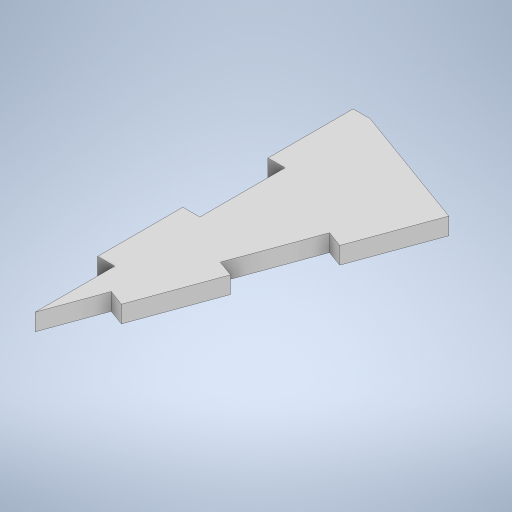
# Autodesk Inventor part: do_sensor_2
Saved by Autodesk Inventor 2023 (Build 270158000, 158)
## iProperties
Created: 2022-11-21
Part Number: do_sensor_2
Material: Generic
Document SubType Name: Modeling
Designer: ADMIN
Density: 1 g/cm^3
Appearance: Default
Author: ADMIN
Autodesk Inventor part; units mm, degrees
ref_plane "YZ Plane" through (0, 0, 0) normal (1, 0, 0) x (0, 1, 0)
ref_plane "XZ Plane" through (0, 0, 0) normal (0, 1, 0) x (-1, 0, 0)
ref_plane "XY Plane" through (0, 0, 0) normal (0, 0, 1) x (1, 0, 0)
sketch "Sketch1" plane through (0, 0, 0) normal (0, 1, 0) x (-1, 0, 0)
  line L0 (-13.5, -14) -> (-32.4622, -7.0983)
  line L1 (-13.5, -14) -> (-10.5, -14)
  line L2 (-10.5, -14) -> (-10.5, 1)
  line L3 (-10.5, 1) -> (-13.5, 1)
  line L4 (-13.5, 1) -> (-13.5, 16)
  line L5 (-13.5, 16) -> (-10.5, 16)
  line L6 (-10.5, 16) -> (-10.5, 31)
  line L7 (-10.5, 31) -> (-13.5, 31)
  line L8 (-13.5, 45) -> (-13.5, 31)
  line L9 (-13.5, 16) -> (-13.5, 1)
  line L10 (-32.4622, -7.0983) -> (-35.2813, -6.0723)
  line L11 (-35.2813, -6.0723) -> (-30.151, 8.0231)
  line L12 (-30.151, 8.0231) -> (-27.3319, 6.9971)
  line L13 (-27.3319, 6.9971) -> (-22.2016, 21.0925)
  line L14 (-22.2016, 21.0925) -> (-25.0207, 22.1185)
  line L15 (-25.0207, 22.1185) -> (-19.8904, 36.2139)
  line L16 (-19.8904, 36.2139) -> (-17.0713, 35.1879)
  line L17 (-13.5, 45) -> (-17.0713, 35.1879)
  line L18 (-22.2016, 21.0925) -> (-27.3319, 6.9971)
  point P0 (0, 0)
  dimension "d0" = 3
  dimension "d1" = 15
  dimension "d2" = 15
  dimension "d3" = 15
  dimension "d4" = 15
  dimension "d5" = 15
  dimension "d6" = 15
  dimension "d7" = 2.8191
  constraints: 38 end point, 14 perpendicular, 2 point on line, 1 vertical
  measures "d0" distance of L0.start L1.end
  measures "d1" distance of L1.end L3.start
  measures "d2" distance of L4.start L5.start
  measures "d3" distance of L5.end L7.start
  measures "d4" distance of L11.start L12.start
  measures "d5" distance of L13.start L14.start
  measures "d6" distance of L14.end L15.end
  measures "d7" horizontal distance of L12.start L13.start
extrude "Extrusion1" add sketch "Sketch1" along normal blind 3
body "Solid1"
